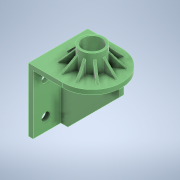
# Autodesk Inventor part: P01_Marcos_Uriel_Martinez_Ortiz3
Saved by Autodesk Inventor 2021 (Build 250183000, 183)
## iProperties
Created: 2021-03-12
Part Number: P01_Marcos_Uriel_Martinez_Ortiz3
Material: Steel ASTM A36
Document SubType Name: Modeling
Designer: uriel
Density: 7.85 g/cm^3
Appearance: Smooth - Dark Forest Green
Mass: 25278.8 g
Surface Area: 4324.93 cm^2
Volume: 3220.23 cm^3
Author: uriel
Autodesk Inventor part; units mm, degrees
ref_plane "YZ Plane" through (0, 0, 0) normal (1, 0, 0) x (0, 1, 0)
ref_plane "XZ Plane" through (0, 0, 0) normal (0, 1, 0) x (-1, 0, 0)
ref_plane "XY Plane" through (0, 0, 0) normal (0, 0, 1) x (1, 0, 0)
sketch "Sketch1" plane through (0, 0, 0) normal (0, 1, 0) x (-1, 0, 0)
  arc A0 (0, 125) -> (0, -125) centre (0, 0) ccw
  line L0 (0, -125) -> (144, -125)
  line L1 (144, -125) -> (144, 125)
  line L2 (144, 125) -> (0, 125)
  circle A1 centre (0, 0) radius 41
  circle A2 centre (0, 0) radius 50
  dimension "d1" = 125
  dimension "d2" = 144
  dimension "d3" = 82
  dimension "d4" = 100
  constraints: 6 end point, 3 centre point, 3 coincident, 2 perpendicular, 2 point on circle, 1 horizontal
  measures "d1" radius of A0
  measures "d2" distance of L0.start L0.end
  measures "d3" diameter of A1
  measures "d4" diameter of A2
extrude "Extrusion1" add sketch "Sketch1" against normal blind 19 contours L2 L1 L0 A0 | A1 | A2
sketch "Sketch2" plane through (0, 0, 0) normal (0, 1, 0) x (-1, 0, 0)
  circle A0 centre (0, 0) radius 41
  circle A1 centre (0, 0) radius 50
  dimension "d7" = 82
  dimension "d8" = 100
  constraints: 2 centre point, 2 coincident
  measures "d7" diameter of A0
  measures "d8" diameter of A1
extrude "Extrusion2" add sketch "Sketch2" along normal blind 80
sketch "Sketch3" plane through (0, 0, 0) normal (0, 0, 1) x (1, 0, 0)
  line L0 (125, 0) -> (0, 0) projected
  line L1 (125, 0) -> (106, 0)
  line L2 (106, 0) -> (50, 0)
  line L3 (106, 0) -> (50, 56)
  line L4 (50, 0) -> (50, 80) projected
  dimension "d11" = 19
  dimension "d12" = 56
  dimension "d13" = 45
  constraints: 6 end point, 3 point on line
  measures "d11" distance of L0.start L1.end
  measures "d12" distance of L1.end L2.end
  measures "d13" angle of L0 L3
extrude "Extrusion3" add sketch "Sketch3" along normal mid plane 9
pattern_circular "Circular Pattern1" count 10 over 360 about axis through (0, 0, 0) along (0, 1, 0) of "Extrusion3"
sketch "Sketch4" plane through (0, -19, 0) normal (0, -1, 0) x (1, 0, 0)
  line L0 (-144, -125) -> (-144, 125) projected
  line L1 (-144, 125) -> (0, 125) projected
  line L2 (-144, -125) -> (-125, -125)
  line L3 (-125, -125) -> (-125, 125)
  line L4 (-125, 125) -> (-144, 125)
  line L5 (-144, 125) -> (-144, -125)
  point P0 (0, 0)
  dimension "d19" = 19
  constraints: 8 end point, 2 parallel, 1 horizontal, 1 perpendicular, 1 point on line
  measures "d19" distance of L4.end L3.end
extrude "Extrusion4" add sketch "Sketch4" along normal blind 250
sketch "Sketch5" plane through (0, 0, 0) normal (0, 0, 1) x (1, 0, 0)
  line L0 (0, -19) -> (125, -19) projected
  line L1 (125, -19) -> (125, -49)
  line L2 (-125, -19) -> (-125, -269) projected
  line L3 (-125, -269) -> (-95, -269)
  line L4 (-95, -269) -> (125, -49)
  line L5 (0, -19) -> (-125, -19) projected
  line L6 (-125, -269) -> (-125, -19)
  line L7 (-125, -19) -> (125, -19)
  point P0 (0, 0)
  dimension "d22" = 30
  dimension "d23" = 30
  constraints: 10 end point, 2 vertical, 1 collinear, 1 horizontal
  measures "d22" distance of L0.end L1.end
  measures "d23" distance of L2.end L3.end
extrude "Extrusion5" add sketch "Sketch5" along normal mid plane 16
sketch "Sketch6" plane through (0, 0, 0) normal (1, 0, 0) x (0, 1, 0)
  line L0 (-19, 125) -> (-19, 8) projected
  line L1 (-19, 125) -> (-19, 71)
  line L2 (-19, 71) -> (-73, 71)
  circle A0 centre (-73, 71) radius 18
  line L3 (-73, 71) -> (-215, 71)
  circle A1 centre (-215, 71) radius 18
  circle A2 centre (-73, -71) radius 18
  circle A3 centre (-215, -71) radius 18
  point P0 (0, 0)
  dimension "d26" = 54
  dimension "d27" = 54
  dimension "d28" = 36
  dimension "d29" = 142
  dimension "d30" = 36
  dimension "d33" = 142
  constraints: 6 end point, 4 centre point, 2 coincident, 1 horizontal, 1 perpendicular, 1 point on line, 1 vertical, 4 other
  measures "d26" distance of L0.start L1.end
  measures "d27" distance of L1.end L2.end
  measures "d28" diameter of A0
  measures "d29" distance of L3.start L3.end
  measures "d30" diameter of A1
  measures "d33" distance of L3.start A2.centre
extrude "Extrusion6" cut sketch "Sketch6" against normal blind 200
body "Solid1"
